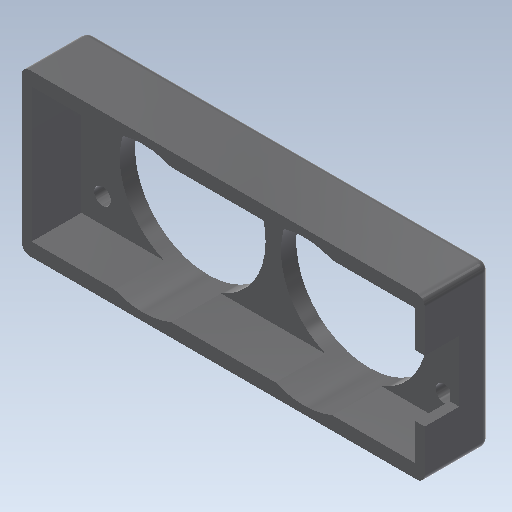
# Autodesk Inventor part: New_Accelite_Controller_Cover_copy
Saved by Autodesk Inventor 2020 (Build 240168000, 168)
## iProperties
Created: 2014-07-12
Part Number: New_Accelite_Controller_Cover_copy
Material: ABS プラスチック
Document SubType Name: Modeling
Designer: andou
Density: 1.06 g/cm^3
Appearance: 滑らか - 標準の灰色
Mass: 3.87174 g
Surface Area: 42.7791 cm^2
Volume: 3.65258 cm^3
Author: andou
Autodesk Inventor part; units mm, degrees
ref_plane "YZ Plane" through (0, 0, 0) normal (1, 0, 0) x (0, 1, 0)
ref_plane "XZ Plane" through (0, 0, 0) normal (0, 1, 0) x (-1, 0, 0)
ref_plane "XY Plane" through (0, 0, 0) normal (0, 0, 1) x (1, 0, 0)
sketch "スケッチ1" plane through (0, 0, 0) normal (0, 0, 1) x (1, 0, 0)
  line L0 (26.25, -10.5) -> (-26.25, -10.5)
  line L1 (-26.25, -10.5) -> (-26.25, 10.5)
  line L2 (-26.25, 10.5) -> (26.25, 10.5)
  line L3 (26.25, 10.5) -> (26.25, -10.5)
  line L4 (26.25, -10.5) -> (-26.25, 10.5) construction
  line L5 (-26.25, -10.5) -> (26.25, 10.5) construction
  point P0 (0, 0)
  dimension "d0" = 52.5
  dimension "d2" = 21
  constraints: 12 end point, 2 midpoint, 2 parallel, 1 horizontal, 1 perpendicular
  measures "d0" distance of L1.end L2.end
  measures "d2" distance of L0.end L1.end
extrude "押し出し1" add sketch "スケッチ1" along normal blind 8.5
sketch "スケッチ19" plane through (0, 0, 0) normal (0, 0, -1) x (-1, 0, 0)
  circle A0 centre (-22.25, 5.5) radius 1.1
  circle A1 centre (22.25, 5.5) radius 1.1
  circle A2 centre (22.25, -5.5) radius 1.1
  circle A3 centre (-22.25, -5.5) radius 1.1
  point P0 (0, 0)
  dimension "d140" = 2.2
  dimension "d141" = 2.2
  dimension "d142" = 2.2
  dimension "d143" = 2.2
  dimension "d144" = 44.5
  dimension "d145" = 22.25
  dimension "d146" = 11
  dimension "d147" = 5.5
  dimension "d148" = 44.5
  dimension "d149" = 11
  constraints: 4 centre point
  measures "d140" diameter of A0
  measures "d141" diameter of A1
  measures "d142" diameter of A2
  measures "d143" diameter of A3
  measures "d144" distance of A1.centre A0.centre
  measures "d145" horizontal distance of point (0, 0) A0.centre
  measures "d146" distance of A3.centre A0.centre
  measures "d147" vertical distance of point (0, 0) A0.centre
  measures "d148" distance of A2.centre A3.centre
  measures "d149" distance of A2.centre A1.centre
extrude "押し出し15" cut sketch "スケッチ19" against normal through all
sketch "スケッチ20" plane through (0, 0, 8.5) normal (0, 0, 1) x (1, 0, 0)
  line L0 (25, -8.75) -> (-25, -8.75)
  line L1 (-25, -8.75) -> (-25, 8.75)
  line L2 (-25, 8.75) -> (25, 8.75)
  line L3 (25, 8.75) -> (25, -8.75)
  point P0 (0, 0)
  dimension "d152" = 50
  dimension "d153" = 25
  dimension "d154" = 17.5
  dimension "d155" = 8.75
  constraints: 8 end point, 2 parallel, 1 horizontal, 1 perpendicular
  measures "d152" distance of L0.start L0.end
  measures "d153" distance from line of L3 point (0, 0)
  measures "d154" distance of L0.end L1.end
  measures "d155" distance from line of L2 point (0, 0)
extrude "押し出し16" cut sketch "スケッチ20" against normal blind 6.5
sketch "スケッチ21" plane through (26.25, -10.5, 0) normal (1, 0, 0) x (0, 0, -1)
  line L0 (-8.5, 0) -> (-8.5, 21) projected
  line L1 (-8.5, 14.5) -> (-4, 14.5)
  line L2 (-4, 14.5) -> (-4, 6.5)
  line L3 (-4, 6.5) -> (-8.5, 6.5)
  line L4 (-8.5, 6.5) -> (-8.5, 14.5)
  line L5 (0, 21) -> (-8.5, 21) projected
  line L6 (0, 0) -> (-8.5, 0) projected
  line L7 (0, 21) -> (0, 0) projected
  point P0 (0, 10.5)
  dimension "d160" = 4
  dimension "d163" = 6.5
  dimension "d164" = 6.5
  constraints: 8 end point, 2 parallel, 1 horizontal, 1 perpendicular, 1 point on line
  measures "d160" distance between parallel lines of L7 L2
  measures "d163" distance between parallel lines of L3 L6
  measures "d164" distance between parallel lines of L5 L1
extrude "押し出し17" cut sketch "スケッチ21" against normal blind 7 contours L0 L1 L2 L3
sketch "スケッチ22" plane through (0, 0, 0) normal (0, 0, -1) x (-1, 0, 0)
  circle A0 centre (10.5, 0) radius 9.5
  circle A1 centre (-10.5, 0) radius 9.5
  point P0 (0, 0)
  dimension "d165" = 19
  dimension "d166" = 19
  dimension "d167" = 10.5
  dimension "d168" = 10.5
  constraints: 2 centre point
  measures "d165" diameter of A0
  measures "d166" diameter of A1
  measures "d167" distance of A0.centre point (0, 0)
  measures "d168" distance of A1.centre point (0, 0)
extrude "押し出し18" cut sketch "スケッチ22" against normal through all
fillet "フィレット3" radius 1 8 edges at (-26.25, 10.5, 4.25) (-26.25, 0, 0) (-26.25, -10.5, 4.25) (0, 10.5, 0) (26.25, 10.5, 4.25) (26.25, 0, 0) (0, -10.5, 0) (26.25, -10.5, 4.25)
